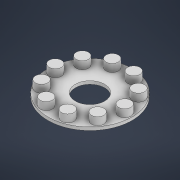
# Autodesk Inventor part: OutputShaft
Saved by Autodesk Inventor 2021 (Build 250183000, 183)
## iProperties
Created: 2022-10-07
Part Number: OutputShaft
Material: Ogólny
Document SubType Name: Modeling
Designer: MicnedSQ
Density: 1 g/cm^3
Appearance: Domyślna
Author: MicnedSQ
Autodesk Inventor part; units mm, degrees
ref_plane "YZ Plane" through (0, 0, 0) normal (1, 0, 0) x (0, 1, 0)
ref_plane "XZ Plane" through (0, 0, 0) normal (0, 1, 0) x (-1, 0, 0)
ref_plane "XY Plane" through (0, 0, 0) normal (0, 0, 1) x (1, 0, 0)
sketch "Szkic3" plane through (0, 0, 0) normal (0, 1, 0) x (-1, 0, 0)
  circle A0 centre (0, 0) radius 27.25
  dimension "d7" = 54.5
  constraints: 1 centre point, 1 coincident
  measures "d7" diameter of A0
extrude "Wyciągnięcie proste3" add sketch "Szkic3" along normal blind 2
sketch "Szkic4" plane through (0, 2, 0) normal (0, 1, 0) x (1, 0, 0)
  circle A0 centre (-22.5, 0) radius 4
  point P0 (0, 0)
  dimension "d10" = 22.5
  dimension "d16" = 8
  constraints: 1 centre point
  measures "d10" distance of point (0, 0) A0.centre
  measures "d16" diameter of A0
extrude "Wyciągnięcie proste4" add sketch "Szkic4" along normal blind 5
pattern_circular "Szyk kołowy1" count 10 over 360 about axis through (0, 0, 0) along (0, 1, 0) of "Wyciągnięcie proste4"
sketch "Szkic5" plane through (0, 0, 0) normal (0, -1, 0) x (1, 0, 0)
  circle A0 centre (22.5, 0) radius 1.85
  point P0 (0, 0)
  dimension "d17" = 3.7
  constraints: 1 centre point, 1 coincident
  measures "d17" diameter of A0
extrude "Wyciągnięcie proste5" cut sketch "Szkic5" against normal blind 6
pattern_circular "Szyk kołowy2" count 5 over 360 about axis through (0, 0, 0) along (0, 1, 0) of "Wyciągnięcie proste5"
sketch "Szkic6" plane through (0, 2, 0) normal (0, 1, 0) x (1, 0, 0)
  circle A0 centre (0, 0) radius 9.5
  dimension "d23" = 19
  constraints: 1 centre point, 1 coincident
  measures "d23" diameter of A0
extrude "Wyciągnięcie proste6" cut sketch "Szkic6" against normal up to surface (2 mm away)
